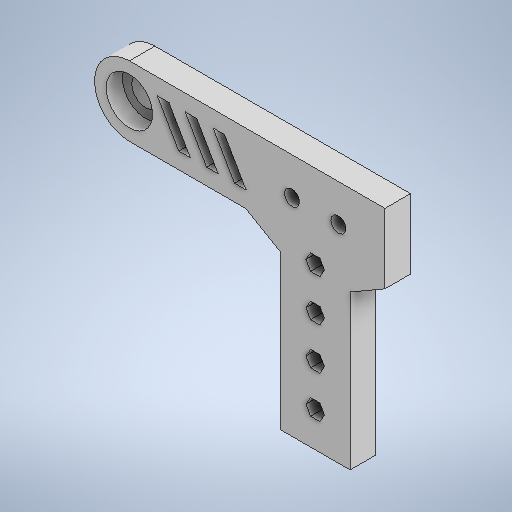
# Autodesk Inventor part: blet_leg_30x30
Saved by Autodesk Inventor 2025 (Build 290162000, 162)
## iProperties
Created: 2024-12-16
Part Number: blet_leg_30x30
Material: Všeobecné
Document SubType Name: Modeling
Designer: lukas
Density: 1 g/cm^3
Appearance: Výchozí
Author: lukas
## iProperties of the stored document blet_leg_30x30_3D tisk.ipt
Created: 2025-01-12
Part Number: blet_leg_30x30_3D tisk
Material: Všeobecné
Document SubType Name: Modeling
Designer: lukas
Density: 1 g/cm^3
Appearance: Výchozí
Author: lukas
Autodesk Inventor part; units mm, degrees
ref_plane "YZ Plane" through (0, 0, 0) normal (1, 0, 0) x (0, 1, 0)
ref_plane "XZ Plane" through (0, 0, 0) normal (0, 1, 0) x (-1, 0, 0)
ref_plane "XY Plane" through (0, 0, 0) normal (0, 0, 1) x (1, 0, 0)
sketch "Náčrt1" plane through (0, 0, 0) normal (0, 0, 1) x (1, 0, 0)
  line L0 (-95, 0) -> (80, 0) projected
  line L1 (0, -73.5) -> (0, 73.5) projected
  line L2 (-55, 52.5) -> (55, 52.5)
  line L3 (55, 52.5) -> (55, 22.5)
  line L4 (55, 22.5) -> (-55, 22.5)
  line L5 (-55, 22.5) -> (-55, 52.5)
  line L6 (40, -52.5) -> (10, -52.5)
  line L7 (10, -52.5) -> (10, 22.5)
  line L8 (10, 22.5) -> (40, 22.5)
  line L9 (40, 22.5) -> (40, -52.5)
  circle A0 centre (-55, 37.5) radius 15
  point P0 (0, 0)
  dimension "d0" = 30
  dimension "d1" = 110
  dimension "d2" = 30
  dimension "d3" = 15
  dimension "d4" = 75
  constraints: 16 end point, 4 parallel, 2 horizontal, 2 perpendicular, 1 midpoint, 1 point on line, 5 other
  measures "d0" distance of L4.end L2.start
  measures "d1" distance of L2.start L2.end
  measures "d2" distance of L6.start L6.end
  measures "d3" distance from line of L3.end L9
  measures "d4" distance of L6.end L7.end
extrude "Vysunutí1" add sketch "Náčrt1" along normal blind 14 contours L7 L4 L9 L0 | L0 L9 L6 L7 | L4 A0 L2 L1 | L1 L2 L3 L4 | A0 L5 | L5 A0
sketch "Náčrt2" plane through (0, 0, 0) normal (0, 0, -1) x (-1, 0, 0)
  line L0 (-55, 52.5) -> (55, 52.5) projected
  line L1 (-55, 52.5) -> (55, 52.5) projected
  line L2 (-55, 22.5) -> (-55, 52.5) projected
  line L3 (-40, 22.5) -> (-55, 22.5) projected
  line L4 (-40, -52.5) -> (-40, 22.5) projected
  line L5 (-10, -52.5) -> (-40, -52.5) projected
  line L6 (-10, 22.5) -> (-10, -52.5) projected
  line L7 (55, 22.5) -> (-10, 22.5) projected
  arc A0 (55, 22.5) -> (55, 52.5) centre (55, 37.5) ccw projected
  point P0 (0, 0)
  constraints: 1 coincident
hole "Díra1" at (-55, 37.5, 0) direction (0, 0, 1) diameter 12 end through all counterbore diameter 20 counterbore depth 7
chamfer "Zkosení1" distance 3 angle 45 8 edges at (0, 52.5, 14) (-70, 37.5, 14) (-22.5, 22.5, 14) (10, -15, 14) (40, -15, 14) (47.5, 22.5, 14) (55, 37.5, 14) (25, -52.5, 14)
sketch "Náčrt3" plane through (0, 0, 14) normal (0, 0, 1) x (1, 0, 0)
  circle A0 centre (-55, 37.5) radius 6 projected
  line L0 (-55, 49.5) -> (52, 49.5) projected
  arc A1 (-55, 49.5) -> (-55, 25.5) centre (-55, 37.5) ccw projected
  line L1 (13, 25.5) -> (-55, 25.5) projected
  line L2 (13, -49.5) -> (13, 25.5) projected
  line L3 (37, -49.5) -> (13, -49.5) projected
  line L4 (37, 25.5) -> (37, -49.5) projected
  line L5 (52, 25.5) -> (37, 25.5) projected
  line L6 (52, 49.5) -> (52, 25.5) projected
  line L7 (0, 73.5) -> (0, -73.5) projected
  line L8 (-95, 0) -> (80, 0) projected
  point P0 (0, 0)
  point P1 (35, 36.5)
  dimension "d17" = 13
  dimension "d18" = 17
  measures "d17" distance from line of L0 point (35, 36.5)
  measures "d18" distance from line of L6 point (35, 36.5)
hole "Díra2" at (35, 36.5, 14) direction (0, 0, -1) diameter 6.5 end through all counterbore diameter 11 counterbore depth 4 clearance for "Strojní šroub se zápustnou hlavou" size "M6" standard "Ansi M metrický profil"
pattern_linear "Obdélníkové pole1" count 2 spacing 20 along (-1, 0, 0) of "Díra2"
sketch "Náčrt4" plane through (0, 0, 14) normal (0, 0, 1) x (1, 0, 0)
  line L0 (-95, 0) -> (80, 0) projected
  line L1 (0, -73.5) -> (0, 73.5) projected
  circle A0 centre (15, 36.5) radius 5.5 projected
  circle A1 centre (35, 36.5) radius 5.5 projected
  circle A2 centre (-55, 37.5) radius 6 projected
  line L2 (-55, 49.5) -> (52, 49.5) projected
  arc A3 (-55, 49.5) -> (-55, 25.5) centre (-55, 37.5) ccw projected
  line L3 (13, 25.5) -> (-55, 25.5) projected
  line L4 (13, -49.5) -> (13, 25.5) projected
  line L5 (37, -49.5) -> (13, -49.5) projected
  line L6 (37, 25.5) -> (37, -49.5) projected
  line L7 (52, 25.5) -> (37, 25.5) projected
  line L8 (52, 49.5) -> (52, 25.5) projected
  line L9 (-33.7624, 29.5) -> (-28.7624, 29.5)
  line L10 (-28.7624, 29.5) -> (-38, 45.5)
  line L11 (-28.7624, 29.5) -> (-10.2872, 29.5) construction
  line L12 (-33.7624, 29.5) -> (-43, 45.5)
  line L13 (-43, 45.5) -> (-38, 45.5)
  point P0 (0, 0)
  dimension "d29" = 120
  dimension "d31" = 5
  dimension "d32" = 4
  dimension "d33" = 4
  dimension "d34" = 12
  constraints: 10 end point, 3 horizontal, 1 equal length, 1 parallel
  measures "d29" angle of L11 L10
  measures "d31" distance of L12.end L10.end
  measures "d32" distance between parallel lines of L2 L13
  measures "d33" distance between parallel lines of L3 L9
  measures "d34" horizontal distance of A2.centre L12.end
extrude "Vysunutí2" cut sketch "Náčrt4" against normal through all contours L12 L13 L10 L9
chamfer "Zkosení2" distance 1 angle 45 4 edges at (-38.3812, 37.5, 14) (-40.5, 45.5, 14) (-33.3812, 37.5, 14) (-31.2624, 29.5, 14)
pattern_linear "Obdélníkové pole2" count 3 spacing 12 along (1, 0, 0) of "Vysunutí2", "Zkosení2"
sketch "Náčrt5" plane through (0, 0, 14) normal (0, 0, 1) x (1, 0, 0)
  line L0 (-32.7321, 46.5) -> (-22.3397, 28.5) projected
  line L1 (-25.4226, 46.5) -> (-32.7321, 46.5) projected
  line L2 (-15.0303, 28.5) -> (-25.4226, 46.5) projected
  line L3 (-22.3397, 28.5) -> (-15.0303, 28.5) projected
  line L4 (-55, 49.5) -> (52, 49.5) projected
  arc A0 (-55, 49.5) -> (-55, 25.5) centre (-55, 37.5) ccw projected
  line L5 (13, 25.5) -> (-55, 25.5) projected
  line L6 (13, -49.5) -> (13, 25.5) projected
  line L7 (37, -49.5) -> (13, -49.5) projected
  line L8 (37, 25.5) -> (37, -49.5) projected
  line L9 (52, 25.5) -> (37, 25.5) projected
  line L10 (52, 49.5) -> (52, 25.5) projected
  circle A1 centre (-55, 37.5) radius 6 projected
  circle A2 centre (35, 36.5) radius 5.5 projected
  circle A3 centre (15, 36.5) radius 5.5 projected
  line L11 (-27.0303, 28.5) -> (-37.4226, 46.5) projected
  line L12 (-34.3397, 28.5) -> (-27.0303, 28.5) projected
  line L13 (-44.7321, 46.5) -> (-34.3397, 28.5) projected
  line L14 (-37.4226, 46.5) -> (-44.7321, 46.5) projected
  line L15 (-20.7321, 46.5) -> (-10.3397, 28.5) projected
  line L16 (-13.4226, 46.5) -> (-20.7321, 46.5) projected
  line L17 (-3.0303, 28.5) -> (-13.4226, 46.5) projected
  line L18 (-10.3397, 28.5) -> (-3.0303, 28.5) projected
  line L19 (0, -73.5) -> (0, 73.5) projected
  line L20 (27, 19.9641) -> (29, 16.5)
  line L21 (29, 16.5) -> (27, 13.0359)
  line L22 (27, 13.0359) -> (23, 13.0359)
  line L23 (23, 13.0359) -> (21, 16.5)
  line L24 (21, 16.5) -> (23, 19.9641)
  line L25 (23, 19.9641) -> (27, 19.9641)
  point P0 (0, 0)
  point P1 (25, 16.5)
  dimension "d43" = 4
  dimension "d44" = 9
  dimension "d45" = 12
  dimension "d52" = 3.4641
  constraints: 12 end point, 13 other
  measures "d43" distance of L24.end L20.start
  measures "d44" distance from line of L9 point (25, 16.5)
  measures "d45" distance from line of L8 point (25, 16.5)
  measures "d52" vertical distance of L23.end L24.end
extrude "Vysunutí3" cut sketch "Náčrt5" against normal through all contours L20 L21 L22 L23 L24 L25
chamfer "Zkosení3" distance 1 angle 45 6 edges at (25, 19.9641, 14) (28, 18.2321, 14) (28, 14.7679, 14) (25, 13.0359, 14) (22, 14.7679, 14) (22, 18.2321, 14)
pattern_linear "Obdélníkové pole3" count 4 spacing 18 along (0, -1, 0) of "Vysunutí3", "Zkosení3"
ref_plane "Pracovní rovina1" through (0, 0, 0) normal (0, 0, -1) x (-1, 0, 0)
sketch "Náčrt7" plane through (0, 0, 0) normal (0, 0, -1) x (-1, 0, 0)
  line L0 (-29, -37.5) -> (-27, -34.0359) projected
  line L1 (-27, -34.0359) -> (-23, -34.0359) projected
  line L2 (-23, -34.0359) -> (-21, -37.5) projected
  line L3 (-21, -37.5) -> (-23, -40.9641) projected
  line L4 (-23, -40.9641) -> (-27, -40.9641) projected
  line L5 (-27, -40.9641) -> (-29, -37.5) projected
  line L6 (-29, -19.5) -> (-27, -16.0359) projected
  line L7 (-27, -16.0359) -> (-23, -16.0359) projected
  line L8 (-23, -16.0359) -> (-21, -19.5) projected
  line L9 (-21, -19.5) -> (-23, -22.9641) projected
  line L10 (-23, -22.9641) -> (-27, -22.9641) projected
  line L11 (-27, -22.9641) -> (-29, -19.5) projected
  line L12 (-29, -1.5) -> (-27, 1.9641) projected
  line L13 (-27, 1.9641) -> (-23, 1.9641) projected
  line L14 (-23, 1.9641) -> (-21, -1.5) projected
  line L15 (-21, -1.5) -> (-23, -4.9641) projected
  line L16 (-23, -4.9641) -> (-27, -4.9641) projected
  line L17 (-27, -4.9641) -> (-29, -1.5) projected
  line L18 (-21, 16.5) -> (-23, 13.0359) projected
  line L19 (-23, 13.0359) -> (-27, 13.0359) projected
  line L20 (-27, 13.0359) -> (-29, 16.5) projected
  line L21 (-29, 16.5) -> (-27, 19.9641) projected
  line L22 (-27, 19.9641) -> (-23, 19.9641) projected
  line L23 (-23, 19.9641) -> (-21, 16.5) projected
  line L24 (19, 45.5) -> (9.7624, 29.5) projected
  line L25 (9.7624, 29.5) -> (4.7624, 29.5) projected
  line L26 (4.7624, 29.5) -> (14, 45.5) projected
  line L27 (14, 45.5) -> (19, 45.5) projected
  line L28 (31, 45.5) -> (21.7624, 29.5) projected
  line L29 (21.7624, 29.5) -> (16.7624, 29.5) projected
  line L30 (16.7624, 29.5) -> (26, 45.5) projected
  line L31 (26, 45.5) -> (31, 45.5) projected
  line L32 (28.7624, 29.5) -> (38, 45.5) projected
  line L33 (38, 45.5) -> (43, 45.5) projected
  line L34 (43, 45.5) -> (33.7624, 29.5) projected
  line L35 (33.7624, 29.5) -> (28.7624, 29.5) projected
  circle A0 centre (-15, 36.5) radius 3.25 projected
  circle A1 centre (-35, 36.5) radius 3.25 projected
  circle A2 centre (55, 37.5) radius 10 projected
  line L36 (-55, 52.5) -> (55, 52.5) projected
  line L37 (-55, 22.5) -> (-55, 52.5) projected
  line L38 (-40, 22.5) -> (-55, 22.5) projected
  line L39 (-40, -52.5) -> (-40, 22.5) projected
  line L40 (-10, -52.5) -> (-40, -52.5) projected
  line L41 (-10, 22.5) -> (-10, -52.5) projected
  line L42 (55, 22.5) -> (-10, 22.5) projected
  arc A3 (55, 22.5) -> (55, 52.5) centre (55, 37.5) ccw projected
  line L43 (-40, 13.8397) -> (-55, 22.5)
  line L44 (-10, 13.8397) -> (5, 22.5)
  line L45 (-10, 22.5) -> (-10, -52.5) projected
  line L46 (-10, 13.8397) -> (-10, 22.5)
  line L47 (-10, 22.5) -> (5, 22.5)
  line L48 (-40, -52.5) -> (-40, 22.5) projected
  line L49 (-40, 13.8397) -> (-40, 22.5)
  line L50 (-40, 22.5) -> (-55, 22.5)
  point P0 (0, 0)
  dimension "d68" = 15
  dimension "d69" = 15
  dimension "d70" = 30
  dimension "d71" = 30
  constraints: 12 end point, 4 collinear, 4 point on line
  measures "d68" distance of L38.start L43.end
  measures "d69" distance of L41.start L44.end
  measures "d70" angle of L42 L44
  measures "d71" angle of L38 L43
extrude "Vysunutí4" add sketch "Náčrt7" against normal blind 11 contours L38 L39 L43 | L44 L41 L42
mirror "Zrcadlit1" about plane through (0, 0, 0) normal (0, 0, 1) remove original yes
